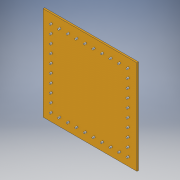
# Autodesk Inventor part: connection_plate
Saved by Autodesk Inventor 2019 (Build 230136000, 136)
## iProperties
Created: 2018-07-11
Part Number: connection_plate
Material: Generic
Document SubType Name: Modeling
Designer: User
Density: 1 g/cm^3
Appearance: Default
Author: User
Autodesk Inventor part; units mm, degrees
ref_plane "YZ Plane" through (0, 0, 0) normal (1, 0, 0) x (0, 1, 0)
ref_plane "XZ Plane" through (0, 0, 0) normal (0, 1, 0) x (-1, 0, 0)
ref_plane "XY Plane" through (0, 0, 0) normal (0, 0, 1) x (1, 0, 0)
sketch "Sketch1" plane through (0, 0, 0) normal (0, 0, 1) x (1, 0, 0)
  line L0 (-358.775, -358.775) -> (358.775, -358.775)
  line L1 (358.775, -358.775) -> (358.775, 358.775)
  line L2 (358.775, 358.775) -> (-358.775, 358.775)
  line L3 (-358.775, 358.775) -> (-358.775, -358.775)
  line L4 (-358.775, -358.775) -> (358.775, 358.775) construction
  line L5 (358.775, -358.775) -> (-358.775, 358.775) construction
  point P0 (0, 0)
  dimension "d0" = 717.55
  dimension "d1" = 717.55
  constraints: 12 end point, 2 midpoint, 2 parallel, 1 horizontal, 1 perpendicular
  measures "d0" distance of L1.end L2.end
  measures "d1" distance of L0.end L1.end
extrude "Extrusion1" add sketch "Sketch1" along normal blind 12.7
sketch "Sketch2" plane through (0, 0, 12.7) normal (0, 0, 1) x (1, 0, 0)
  circle A0 centre (-293.5432, -293.5432) radius 6.35
  line L0 (-358.775, 358.775) -> (-358.775, -358.775) projected
  line L1 (-293.5432, -293.5432) -> (293.5432, -293.5432)
  line L2 (293.5432, -293.5432) -> (293.5432, 293.5432)
  line L3 (293.5432, 293.5432) -> (-293.5432, 293.5432)
  line L4 (-293.5432, 293.5432) -> (-293.5432, -293.5432)
  line L5 (-293.5432, -293.5432) -> (293.5432, 293.5432) construction
  line L6 (293.5432, -293.5432) -> (-293.5432, 293.5432) construction
  point P0 (0, 0)
  dimension "d4" = 12.7
  dimension "d6" = 587.0864
  constraints: 12 end point, 2 midpoint, 2 parallel, 2 perpendicular, 1 centre point, 1 coincident, 1 horizontal
  measures "d4" diameter of A0
  measures "d6" distance of L3.end L1.start
extrude "Extrusion2" add sketch "Sketch2" along normal blind 12.7 contours L1 L4 A0 | A0 L4 L1
pattern_linear "Rectangular Pattern1" count 10 spacing 65.2318 along (1, 0, 0) of "Extrusion2"
pattern_linear "Rectangular Pattern2" count 10 spacing 65.2318 along (0, 1, 0) of "Extrusion2"
ref_plane "Work Plane1" through (-358.775, 358.775, 0) normal (0.7071068, 0.7071068, 0) x (0, 0, 1)
mirror "Mirror1" about plane through (-358.775, 358.775, 0) normal (0.7071068, 0.7071068, 0) of "Extrusion2", "Rectangular Pattern1", "Rectangular Pattern2"
body "Solid1"
